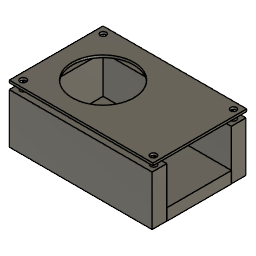
box for hfcv (Autodesk Fusion 360 design; units mm, degrees)
part number: 2025-12-04-16-13-48-597
Autodesk Fusion 360 part; units mm, degrees
sketch "Sketch1" plane through (0, 0, 0) normal (0, 0, 1) x (1, 0, 0)
  line L0 (0, 0) -> (48.7101, 0)
  line L1 (48.7101, 0) -> (48.7101, 32)
  line L2 (48.7101, 32) -> (0, 32)
  line L3 (0, 32) -> (0, 0)
  line L4 (5, 27) -> (48.76, 27)
  line L5 (48.76, 27) -> (48.76, 5)
  line L6 (48.76, 5) -> (5, 5)
  line L7 (5, 5) -> (5, 27)
  circle A0 centre (16, 16) radius 10.5
  line L8 (16, 16) -> (16, 27) construction
  line L9 (16, 16) -> (16, 5) construction
  circle A1 centre (2.3717, 29.6206) radius 1
  circle A2 centre (46.8313, 29.5894) radius 1
  line L10 (0, 16) -> (48.76, 16) construction
  circle A3 centre (2.3717, 2.3794) radius 1
  circle A4 centre (46.8313, 2.4106) radius 1
  dimension "d1" = 5
  dimension "d2" = 5
  dimension "d4" = 43.76
  dimension "d6" = 5
  dimension "d7" = 22
  dimension "d8" = 21
  dimension "d9" = 11
  dimension "d14" = 2
  dimension "d15" = 2
  constraint horizontal L0
  constraint vertical L1
  constraint horizontal L2
  constraint vertical L3
  constraint coincident L0.start L3.end
  constraint horizontal L4
  constraint vertical L5
  constraint horizontal L6
  constraint vertical L7
  constraint coincident A0.centre L8.start
  constraint coincident L4 L8.end
  constraint perpendicular L4 L8
  constraint coincident L6 L9.end
  constraint perpendicular L6 L9
  constraint equal L8 L9
  constraint midpoint L3 L10.start
  constraint midpoint L5 L10.end
  constraint symmetric A1 L10 A3
  constraint symmetric A2 L10 A4
  measures "d1" distance of L2 L4
  measures "d2" distance of L0 L6
  measures "d4" distance of L4.start L4.end
  measures "d6" distance of L3 L7
  measures "d7" distance of L4.end L5.end
  measures "d8" diameter of A0
  measures "d9" distance of L7 A0.centre
  measures "d14" diameter of A1
  measures "d15" diameter of A2
extrude "Extrude1" add sketch "Sketch1" along normal blind 17 contours L0 L1 L2 L3 L4 L6 L7 | A1 | A2 | A3 | A4 makes body 1
extrude "Extrude2" add sketch "Sketch1" along normal blind 4 contours L1 L4 L6 L7 | L1 L4 L5 L6 | A0 bodies 1
extrude "Extrude3" cut sketch "Sketch1" along normal blind 15 from surface at 11 contours A1 | A2 | A3 | A4 bodies 1
ref_plane "WorkPlane1" through (0, 0, 19) normal (0, 0, 1) x (1, 0, 0)
sketch "Sketch2" plane through (0, 0, 19) normal (0, 0, 1) x (1, 0, 0)
  line L0 (0, 32) -> (49, 32)
  line L1 (49, 32) -> (49, 0)
  line L2 (49, 0) -> (0, 0)
  line L3 (0, 0) -> (0, 32)
  circle A0 centre (2.4192, 29.6507) radius 1.0096
  circle A1 centre (46.8253, 29.6507) radius 1.0172
  circle A2 centre (2.4192, 2.362) radius 1.0849
  circle A3 centre (46.8253, 2.362) radius 1.0543
  constraint horizontal L0
  constraint vertical L1
  constraint horizontal L2
  constraint vertical L3
extrude "Extrude4" add sketch "Sketch2" along normal blind 0.8 separate body contours L0 L1 L2 L3 | A0 | A1 | A2 | A3 makes body 2
extrude "Extrude5" cut sketch "Sketch2" along normal blind 5 contours A0 | A1 | A2 | A3 bodies 2
extrude "Extrude6" cut sketch "Sketch1" along normal through all and the other way through all contours A0 bodies 1 2
